Autodesk Inventor part; units mm, degrees
(part 2 of 2)
sketch "Sketch32" plane through (-99.4156, 5.08, 29.4899) normal (-0.7071068, 0, 0.7071068) x (0.7071068, 0, 0.7071068)
  arc A0 (-65.0491, 11.43) -> (-51.5871, 11.43) centre (-58.3181, 11.43) ccw projected
  circle A1 centre (-58.3181, 11.43) radius 54.61
  arc A2 (0, 11.43) -> (-116.6362, 11.43) centre (-58.3181, 11.43) ccw projected
  circle A3 centre (-58.3181, 11.43) radius 58.3181
  line L0 (-116.6362, 0) -> (-116.6362, -5.08) projected
  line L1 (-116.6362, 0) -> (-112.9281, 0)
  line L2 (-112.9281, 0) -> (-112.9281, 11.43)
  line L3 (-112.9281, 11.43) -> (-116.6362, 11.43)
  line L4 (-116.6362, 11.43) -> (-116.6362, 0)
  line L5 (0, 0) -> (0, 11.43) projected
  line L6 (0, 0) -> (-3.7081, 0)
  line L7 (-3.7081, 0) -> (-3.7081, 11.43)
  line L8 (-3.7081, 11.43) -> (0, 11.43)
  line L9 (0, 11.43) -> (0, 0)
  line L10 (-116.6362, 0) -> (0, 0)
  line L11 (0, 0) -> (0, 69.7481)
  line L12 (0, 69.7481) -> (-116.6362, 69.7481)
  line L13 (-116.6362, 69.7481) -> (-116.6362, 0)
  line L14 (-116.6362, 0) -> (-116.6362, 69.7484) projected
  line L15 (-116.6362, 59.9876) -> (0, 59.9876)
  line L16 (0, 59.9876) -> (0, 82.5701)
  line L17 (0, 82.5701) -> (-116.6362, 82.5701)
  line L18 (-116.6362, 82.5701) -> (-116.6362, 59.9876)
  point P0 (49.445, -5.08)
  point P1 (-3.7081, 0)
  point P2 (-112.9281, 0)
  point P3 (-116.6362, 11.43)
  point P4 (-58.3181, 69.7481)
  point P5 (0, 11.43)
  dimension "d153" = 109.22
  constraints: 32 end point, 8 parallel, 4 horizontal, 4 perpendicular, 3 point on line, 2 coincident, 2 point on circle, 1 centre point, 1 horizontal alignment, 2 other
  measures "d153" diameter of A1
extrude "Extrusion30" cut sketch "Sketch32" against normal up to surface (19.3079 mm away) contours A1 L10 L15 | L7 L10 A1 | L15 A1 | A2 L15 L11 | A2 L12 L11 L15 | L10 L2 A1 | L15 L13 L12 A2 | A2 L13 L15 | L12 L18 L17 L16
sketch "Sketch33" plane through (-102.0376, 5.08, 26.8678) normal (-0.7071068, 0, 0.7071068) x (0.7071068, 0, 0.7071068)
  arc A0 (0, 11.43) -> (-109.22, 11.43) centre (-54.61, 11.43) ccw projected
  circle A1 centre (-54.61, 11.43) radius 54.61
  circle A2 centre (-54.61, 11.43) radius 58.3181
  line L0 (-112.9281, 0) -> (-112.9281, 11.43) projected
  line L1 (-103.9478, -5.08) -> (-112.9281, -5.08) projected
  line L2 (-112.9281, 11.43) -> (-109.22, 11.43)
  line L3 (-109.22, 11.43) -> (-109.22, -5.08)
  line L4 (-109.22, -5.08) -> (-112.9281, -5.08)
  line L5 (-112.9281, -5.08) -> (-112.9281, 11.43)
  line L6 (3.7081, 11.43) -> (0, 11.43)
  line L7 (0, 11.43) -> (0, -5.08)
  line L8 (0, -5.08) -> (3.7081, -5.08)
  line L9 (3.7081, -5.08) -> (3.7081, 11.43)
  point P0 (53.1531, -5.08)
  point P1 (-109.22, 11.43)
  point P2 (0, 11.43)
  constraints: 16 end point, 4 parallel, 3 point on line, 2 centre point, 2 coincident, 2 horizontal, 2 perpendicular, 1 point on circle
extrude "Extrusion31" add sketch "Sketch33" against normal up to surface (34.2939 mm away) contours A0 L2 A2 L6 | L6 A2 L8 L7 | L3 L1 A2 L2 | L9 L8 A2 | A2 L1 L5 L0
sketch "Sketch34" plane through (80.2899, 0, -52.9844) normal (0.7071068, 0, 0.7071068) x (0.7071068, 0, -0.7071068)
  arc A0 (-65.0491, 16.51) -> (-51.5871, 16.51) centre (-58.3181, 16.51) ccw projected
  circle A1 centre (-58.3181, 16.51) radius 54.61
  circle A2 centre (-58.3181, 16.51) radius 58.3181
  line L0 (-112.9281, 5.08) -> (-112.9281, 0) projected
  line L1 (-116.6362, 16.51) -> (-112.9281, 16.51)
  line L2 (-112.9281, 16.51) -> (-112.9281, 0)
  line L3 (-112.9281, 0) -> (-116.6362, 0)
  line L4 (-116.6362, 0) -> (-116.6362, 16.51)
  line L5 (-3.7081, 16.51) -> (-3.7081, 0) projected
  line L6 (0, 16.51) -> (-3.7081, 16.51)
  line L7 (-3.7081, 16.51) -> (-3.7081, 0)
  line L8 (-3.7081, 0) -> (0, 0)
  line L9 (0, 0) -> (0, 16.51)
  point P0 (-94.2391, 0)
  point P1 (-112.9281, 5.08)
  point P2 (-112.9281, 16.51)
  constraints: 16 end point, 4 parallel, 2 coincident, 2 horizontal, 2 perpendicular, 2 point on circle, 1 centre point, 2 other
extrude "Extrusion32" add sketch "Sketch34" against normal up to surface (34.2939 mm away) contours L6 A2 L8 L5 | A1 L1 A2 L6 | L2 L0 L3 A2 L1 | L9 L8 A2 | A2 L3 L4
sketch "Sketch35" plane through (0.4379, 5.08, -230.0676) normal (0.7071068, 0, -0.7071068) x (-0.7071068, 0, -0.7071068)
  arc A0 (-61.3407, 11.43) -> (-47.8787, 11.43) centre (-54.6097, 11.43) ccw projected
  circle A1 centre (-54.6097, 11.43) radius 54.6097
  arc A2 (-63.8807, 11.43) -> (-45.3387, 11.43) centre (-54.6097, 11.43) ccw projected
  circle A3 centre (-54.6097, 11.43) radius 58.3181
  line L0 (-109.2197, -5.08) -> (-109.2197, 0) projected
  line L1 (-112.9278, 11.43) -> (-109.2197, 11.43)
  line L2 (-109.2197, 11.43) -> (-109.2197, -5.08)
  line L3 (-109.2197, -5.08) -> (-112.9278, -5.08)
  line L4 (-112.9278, -5.08) -> (-112.9278, 11.43)
  line L5 (0.0003, -5.08) -> (0.0003, 11.43) projected
  line L6 (3.7084, 11.43) -> (0.0003, 11.43)
  line L7 (0.0003, 11.43) -> (0.0003, -5.08)
  line L8 (0.0003, -5.08) -> (3.7084, -5.08)
  line L9 (3.7084, -5.08) -> (3.7084, 11.43)
  line L10 (-181.6807, -5.08) -> (-112.9278, -5.08) projected
  line L11 (-114.206, -5.08) -> (7.9528, -5.08)
  line L12 (-112.9278, 11.43) -> (7.9528, 11.43)
  line L13 (-112.9278, -5.08) -> (-109.2197, -5.08)
  line L14 (-109.2197, -5.08) -> (-109.2197, 11.43)
  line L15 (-109.2197, 11.43) -> (-112.9278, 11.43)
  line L16 (-112.9278, 11.43) -> (-112.9278, -5.08)
  line L17 (3.7084, -5.08) -> (0.0003, -5.08)
  line L18 (0.0003, -5.08) -> (0.0003, 11.43)
  line L19 (0.0003, 11.43) -> (3.7084, 11.43)
  line L20 (3.7084, 11.43) -> (3.7084, -5.08)
  point P0 (-162.3728, -5.08)
  point P1 (0, 11.43)
  point P2 (0.0003, 11.43)
  point P3 (-109.2197, 0)
  point P4 (-109.2197, 11.43)
  point P5 (-109.2194, 11.43)
  constraints: 36 end point, 8 parallel, 5 horizontal, 4 perpendicular, 2 centre point, 2 coincident, 2 point on circle, 2 point on line, 1 collinear
extrude "Extrusion33" add sketch "Sketch35" against normal up to surface (34.2939 mm away) contours L1 A3 L6 A1 | L2 L0 L3 A3 L1 | L6 A3 L8 L5 | A3 L3 L4 | L9 L8 A3
sketch "Sketch36" plane through (-179.2678, 5.08, -152.8376) normal (-0.7071068, 0, -0.7071068) x (-0.7071068, 0, 0.7071068)
  arc A0 (-61.341, 11.43) -> (-47.879, 11.43) centre (-54.61, 11.43) ccw projected
  circle A1 centre (-54.61, 11.43) radius 54.61
  circle A2 centre (-54.61, 11.43) radius 58.3181
  arc A3 (3.7081, 11.43) -> (-112.9281, 11.43) centre (-54.61, 11.43) ccw projected
  line L0 (0, 0) -> (0, -5.08) projected
  line L1 (3.7081, 11.43) -> (0, 11.43)
  line L2 (0, 11.43) -> (0, -5.08)
  line L3 (0, -5.08) -> (3.7081, -5.08)
  line L4 (3.7081, -5.08) -> (3.7081, 11.43)
  line L5 (-109.22, -5.08) -> (-109.22, 0) projected
  line L6 (-112.9281, 11.43) -> (-109.22, 11.43)
  line L7 (-109.22, 11.43) -> (-109.22, -5.08)
  line L8 (-109.22, -5.08) -> (-112.9281, -5.08)
  line L9 (-112.9281, -5.08) -> (-112.9281, 11.43)
  point P0 (-18.689, -5.08)
  point P1 (0, 11.43)
  point P2 (0, 0)
  point P3 (-109.22, 11.43)
  constraints: 16 end point, 4 parallel, 2 centre point, 2 coincident, 2 horizontal, 2 perpendicular, 1 point on circle, 1 point on line
extrude "Extrusion34" add sketch "Sketch36" against normal up to surface (34.2939 mm away) contours A1 L6 A2 L1 | L1 A2 L3 L0 L2 | L7 L5 L8 A2 L6 | L4 L3 A2 | A2 L8 L9
sketch "Sketch37" plane through (80.2899, 0, -52.9844) normal (1, 0, 0) x (0, 0, -1)
  line L0 (0, 5.08) -> (0, 16.51) projected
  line L1 (97.2312, 5.08) -> (97.2312, 16.51) projected
  line L2 (0, 5.08) -> (97.2312, 5.08)
  line L3 (97.2312, 5.08) -> (97.2312, 16.51)
  line L4 (97.2312, 16.51) -> (0, 16.51)
  line L5 (0, 16.51) -> (0, 5.08)
  point P0 (-52.9844, 0)
  constraints: 8 end point, 2 parallel, 1 horizontal, 1 perpendicular
extrude "Extrusion35" add sketch "Sketch37" against normal blind 2.54
sketch "Sketch38" plane through (80.2899, 0, -52.9844) normal (1, 0, 0) x (0, 0, -1)
  circle A0 centre (37.3634, 17.78) radius 8.89 projected
  circle A1 centre (37.3634, 17.78) radius 8.89
  line L0 (37.3634, 17.78) -> (37.6174, 17.78)
  circle A2 centre (37.6174, 17.78) radius 8.8936
  line L1 (2.54, 16.51) -> (94.6912, 16.51) projected
  line L2 (48.6156, 16.51) -> (48.6156, 24.543)
  circle A3 centre (59.8678, 17.78) radius 8.89
  circle A4 centre (59.8678, 17.78) radius 8.89
  line L3 (59.8678, 17.78) -> (59.6138, 17.78)
  circle A5 centre (59.6138, 17.78) radius 8.8936
  point P0 (-52.9844, 0)
  dimension "d166" = 0.254
  constraints: 6 end point, 5 centre point, 4 coincident, 4 symmetric about line, 1 horizontal, 1 midpoint, 1 perpendicular, 3 other
  measures "d166" distance of L0.start L0.end
extrude "Extrusion36" cut sketch "Sketch38" against normal blind 2.54 contours A0 L1 A2 | A0 A2 L1 | L1 A2 A0 | A0 A2 L1 | A5 A3 L1 | L1 A3 A5 | A3 A5 L1 | L1 A5 A3 picked at (34.6115, 17.6453) picked at (46.3481, 18.4514) picked at (46.1463, 15.8174) picked at (40.1974, 15.8308) picked at (51.0223, 19.4222) picked at (51.0849, 15.8174) picked at (56.8666, 17.657) picked at (57.0338, 15.8308)
sketch "Sketch39" plane through (-2.1844, 5.08, -232.6899) normal (0, 0, -1) x (-1, 0, 0)
  line L0 (0, 0) -> (0, -5.08) projected
  line L1 (97.2312, 0) -> (97.2312, 11.43) projected
  line L2 (0, 0) -> (97.2312, 0)
  line L3 (97.2312, 0) -> (97.2312, 11.43)
  line L4 (97.2312, 11.43) -> (0, 11.43)
  line L5 (0, 11.43) -> (0, 0)
  circle A0 centre (37.3634, 12.7) radius 8.89 projected
  line L6 (37.3634, 12.7) -> (37.6174, 12.7)
  circle A1 centre (37.6174, 12.7) radius 8.8936
  line L7 (48.6156, 11.43) -> (48.6156, 20.1253)
  circle A2 centre (59.8678, 12.7) radius 8.89
  line L8 (59.8678, 12.7) -> (59.6138, 12.7)
  circle A3 centre (59.6138, 12.7) radius 8.8936
  point P0 (-2.1844, -5.08)
  point P1 (68.4163, 11.43)
  point P2 (50.8113, 11.43)
  point P3 (46.4199, 11.43)
  point P4 (28.8149, 11.43)
  dimension "d169" = 0.254
  constraints: 14 end point, 3 centre point, 3 symmetric about line, 2 coincident, 2 horizontal, 2 parallel, 1 midpoint, 1 perpendicular, 1 vertical, 2 other
  measures "d169" distance of L6.start L6.end
extrude "Extrusion37" add sketch "Sketch39" against normal blind 2.54 contours L2 L5 L4 A0 A1 A3 A2 L1 | A2 A3 L4 | L4 A1 A0 picked at (68.4008, 10.7507) picked at (28.8304, 10.7507)
sketch "Sketch40" plane through (0, 5.08, 0) normal (0, 1, 0) x (1, 0, 0)
  line L0 (-77.0439, 7.4399) -> (-24.6342, 7.4399)
  line L1 (-24.6342, 7.4399) -> (-24.6342, -1.5706)
  line L2 (-24.6342, -1.5706) -> (-77.0439, -1.5706)
  line L3 (-77.0439, -1.5706) -> (-77.0439, 7.4399)
  line L4 (-77.0439, 204.4692) -> (-24.6342, 204.4692)
  line L5 (-24.6342, 204.4692) -> (-24.6342, 196.1992)
  line L6 (-24.6342, 196.1992) -> (-77.0439, 196.1992)
  line L7 (-77.0439, 196.1992) -> (-77.0439, 204.4692)
  line L8 (51.7889, 127.7769) -> (45.2093, 127.7769)
  line L9 (45.2093, 127.7769) -> (45.2093, 74.9344)
  line L10 (45.2093, 74.9344) -> (51.7889, 74.9344)
  line L11 (51.7889, 74.9344) -> (51.7889, 127.7769)
  point P0 (0, 0)
  constraints: 24 end point, 6 parallel, 3 horizontal, 3 perpendicular, 2 point on line
extrude "Extrusion38" cut sketch "Sketch40" along normal through all
sketch "Sketch41" plane through (-2.1844, 0, 29.4899) normal (0, 0, 1) x (1, 0, 0)
  line L0 (-97.2312, 0) -> (-97.2312, 16.51) projected
  line L1 (0, 16.51) -> (0, 5.08) projected
  line L2 (-97.2312, 16.51) -> (0, 16.51)
  line L3 (0, 16.51) -> (0, 5.08)
  line L4 (0, 5.08) -> (-97.2312, 5.08)
  line L5 (-97.2312, 5.08) -> (-97.2312, 16.51)
  arc A0 (-68.4163, 16.51) -> (-50.8113, 16.51) centre (-59.6138, 17.78) ccw projected
  circle A1 centre (-59.6138, 17.78) radius 8.8936
  arc A2 (-46.4199, 16.51) -> (-28.8149, 16.51) centre (-37.6174, 17.78) ccw projected
  circle A3 centre (-37.6174, 17.78) radius 8.8936
  point P0 (2.1844, 0)
  constraints: 8 end point, 2 centre point, 2 coincident, 2 parallel, 1 horizontal, 1 perpendicular
extrude "Extrusion39" add sketch "Sketch41" against normal blind 2.54 contours L0 L2 A0 A2 L1 L4
body "Solid1"
